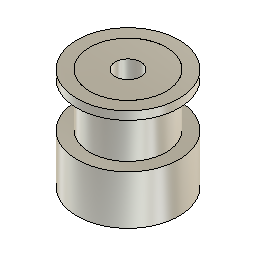
Pulley, 20 tooths, drill hole 4mm (Autodesk Fusion 360 design; units mm, degrees)
Autodesk Fusion 360 part; units mm, degrees
sketch "Skizze1" plane through (0, 0, 0) normal (0, 0, 1) x (1, 0, 0)
  circle A0 centre (0, 0) radius 8
  circle A1 centre (0, 0) radius 2
  dimension "d1" = 16
  dimension "d2" = 4
  constraint coincident A0.centre A1.centre
  constraint concentric A0 A1
  measures "d1" diameter of A0
  measures "d2" diameter of A1
extrude "Extrusion1" add sketch "Skizze1" along normal blind 7.7 makes body 1
sketch "Skizze2" plane through (0, 0, 7.7) normal (0, 0, 1) x (-1, 0, 0)
  circle A0 centre (0, 0) radius 2
  circle A1 centre (0, 0) radius 8
  circle A2 centre (0, 0) radius 2
  circle A3 centre (0, 0) radius 6
  dimension "d5" = 4
  dimension "d6" = 12
  constraint coincident A0.centre A1.centre
  constraint concentric A2 A3
  measures "d5" diameter of A2
  measures "d6" diameter of A3
extrude "Extrusion2" add sketch "Skizze2" along normal blind 7 contours A3 bodies 1
sketch "Skizze3" plane through (0, 0, 14.7) normal (0, 0, 1) x (-1, 0, 0)
  circle A0 centre (0, 0) radius 2
  circle A1 centre (0, 0) radius 6
  circle A2 centre (0, 0) radius 2
  circle A3 centre (0, 0) radius 8
  dimension "d9" = 4
  dimension "d10" = 16
  constraint concentric A0 A2
  constraint coincident A0.centre A1.centre
  measures "d9" diameter of A2
  measures "d10" diameter of A3
extrude "Extrusion4" add sketch "Skizze3" along normal blind 1.3 separate body contours A3 makes body 2
extrude "Extrusion3" add sketch "Skizze3" along normal blind 1.3 contours A1 bodies 1
